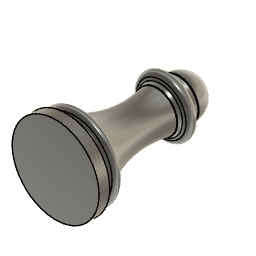
pon (Autodesk Fusion 360 design; units mm, degrees)
Autodesk Fusion 360 part; units mm, degrees
sketch "Szkic1" plane through (0, 0, 0) normal (0, 0, 1) x (1, 0, 0)
  line L0 (13, 5.5) -> (13, 0) construction
  arc A0 (5.7937, 40.0916) -> (6.2088, 39.5139) centre (6.1498, 39.9095) ccw
  arc A1 (8.5637, 36.5139) -> (7.7385, 36.0788) centre (8.5637, 35.5139) ccw
  arc A2 (6.9813, 34.9183) -> (10.8247, 10.2679) centre (41.581, 27.6882) ccw
  arc A3 (6.9824, 42.5042) -> (0, 50) centre (0, 43) ccw
  line L1 (0, 47.5) -> (0, 50)
  line L2 (8.5637, 38.0139) -> (10.0637, 38.0139)
  line L3 (0, 0) -> (15, 0)
  line L4 (0, 0) -> (13, 0) construction
  arc A4 (13, 6.5) -> (13, 9) centre (13, 7.75) ccw
  arc A5 (13, 6.5) -> (12.6552, 4.5613) centre (13, 5.5) ccw
  line L5 (8.5637, 38.0139) -> (8.5637, 35.5139) construction
  line L6 (15, 0) -> (15, 3.7)
  line L7 (15, 3.7) -> (12.6552, 4.5613)
  arc A6 (7.0428, 35.0624) -> (6.9813, 34.9183) centre (7.3728, 34.8365) ccw
  arc A7 (10.8247, 10.2679) -> (13, 9) centre (13, 11.5) ccw
  line L8 (0, 0) -> (0, 47.5)
  line L9 (13, 5.5) -> (13, 16.9401) construction
  line L10 (7.0428, 35.0624) -> (7.7385, 36.0788)
  arc A8 (6.9289, 42.312) -> (6.9824, 42.5042) centre (6.4837, 42.5396) ccw
  line L11 (5.7937, 40.0916) -> (6.9289, 42.312)
  line L12 (4, 34) -> (0, 34) construction
  arc A9 (8.5637, 36.5139) -> (8.5637, 39.5139) centre (8.5637, 38.0139) ccw
  line L13 (8.5637, 39.5139) -> (6.0909, 39.5139)
  dimension "d78" = 15
  dimension "d79" = 3.7
  dimension "d80" = 4
  dimension "d81" = 2
  dimension "d82" = 2.5
  dimension "d83" = 13
  dimension "d84" = 43
  dimension "d85" = 5
  dimension "d86" = 2
  dimension "d87" = 0.8
  dimension "d88" = 3
  dimension "d89" = 7
  dimension "d90" = 2.5
  dimension "d91" = 0.4
  dimension "d92" = 0.5
  dimension "d93" = 5.5
  constraint coincident L3.start L4.start
  constraint horizontal L3
  constraint perpendicular L3 L6
  constraint perpendicular L3 L8
  constraint coincident L12.end L8
  constraint perpendicular L8 L12
  constraint tangent A5 L7
  constraint tangent A4 A5
  constraint coincident L0.end L3
  constraint coincident L0.start A5.centre
  constraint parallel L1 L8
  constraint parallel L0 L9
  constraint coincident A7.centre L9
  constraint tangent A0 L11
  constraint coincident A0.end L13
  constraint coincident L13.end A0
  constraint tangent A9 L13
  constraint coincident L2.start L5.start
  constraint coincident A1.centre L5.end
  constraint vertical L5
  constraint tangent A1 L10
  constraint coincident A1.start L5
  constraint tangent A6 L10
  constraint tangent A2 A6
  constraint tangent A3 A8
  constraint tangent A8 L11
  constraint coincident L2.end A9
  constraint perpendicular L2 L5
  constraint vertical L9
  constraint coincident A4.centre L9
  constraint tangent A4 A7
  constraint tangent A2 A7
  measures "d78" distance of L3.start L3.end
  measures "d79" distance of L3.end L6.end
  measures "d80" distance of L12.start L12.end
  measures "d81" diameter of A5
  measures "d82" diameter of A4
  measures "d83" distance of L3.start L0.end
  measures "d84" distance of L3.start A3.centre
  measures "d85" diameter of A7
  measures "d86" diameter of A1
  measures "d87" diameter of A0
  measures "d88" diameter of A9
  measures "d89" radius of A3
  measures "d90" distance of L2.start A1.centre
  measures "d91" radius of A6
  measures "d92" radius of A8
  measures "d93" vertical distance of L0.start L3.end
revolve "Obrót1" add sketch "Szkic1" angle 360 about axis through (0, 0, 0) along (0, 1, 0)
equation "d7 = 2 mm"
equation "d10 = 3 mm"
equation "d25 = 14 mm"
equation "d80 = d10 + d7 / 2"
equation "d84 = 50 mm - d25 / 2"
